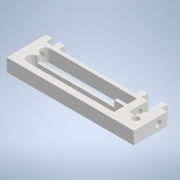
# Autodesk Inventor part: bottom slot
Saved by Autodesk Inventor 2020 (Build 240168000, 168)
## iProperties
Created: 2019-11-08
Part Number: bottom slot
Material: Generic
Document SubType Name: Modeling
Designer: Hymowitz
Density: 1 g/cm^3
Appearance: Default
Author: Hymowitz
## iProperties of the stored document _3DPrint.ipt
Created: 2019-11-25
Part Number: _3DPrint
Material: Generic
Document SubType Name: Modeling
Designer: Hymowitz
Density: 1 g/cm^3
Appearance: Default
Author: Hymowitz
Autodesk Inventor part; units mm, degrees
ref_plane "YZ Plane" through (0, 0, 0) normal (1, 0, 0) x (0, 1, 0)
ref_plane "XZ Plane" through (0, 0, 0) normal (0, 1, 0) x (-1, 0, 0)
ref_plane "XY Plane" through (0, 0, 0) normal (0, 0, 1) x (1, 0, 0)
sketch "Sketch1" plane through (0, 0, 0) normal (0, 1, 0) x (-1, 0, 0)
  line L0 (31.75, -3.048) -> (-31.75, -3.048)
  line L1 (-31.75, -3.048) -> (-31.75, 0)
  line L2 (-31.75, 0) -> (31.75, 0)
  line L3 (31.75, 0) -> (31.75, -3.048)
  line L4 (-31.75, 0) -> (31.75, 0)
  line L5 (31.75, 0) -> (31.75, 16.5722)
  line L6 (31.75, 16.5722) -> (-31.75, 16.5722)
  line L7 (-31.75, 16.5722) -> (-31.75, 0)
  line L8 (24.7167, 10.8097) -> (-19.6375, 10.8097) construction
  line L9 (24.7167, 13.3972) -> (-19.6375, 13.3972)
  line L10 (-19.6375, 8.2222) -> (24.7167, 8.2222)
  arc A0 (24.7167, 8.2222) -> (24.7167, 13.3972) centre (24.7167, 10.8097) ccw
  arc A1 (-19.6375, 13.3972) -> (-19.6375, 8.2222) centre (-19.6375, 10.8097) ccw
  line L11 (24.7167, 4.2534) -> (-24.7167, 4.2534) construction
  line L12 (24.7167, 6.6347) -> (-24.7167, 6.6347)
  line L13 (-24.7167, 1.8722) -> (24.7167, 1.8722)
  arc A2 (24.7167, 1.8722) -> (24.7167, 6.6347) centre (24.7167, 4.2534) ccw
  arc A3 (-24.7167, 6.6347) -> (-24.7167, 1.8722) centre (-24.7167, 4.2534) ccw
  line L14 (0, 0) -> (0, 22.7513) construction
  circle A4 centre (-26.9875, 10.8097) radius 1.5875
  point P0 (0, 4.2534)
  dimension "d5" = 49.4334
  dimension "d6" = 5.175
  dimension "d7" = 4.7625
  dimension "d8" = 4.2534
  dimension "d23" = 7.0333
  dimension "d24" = 3.175
  dimension "d25" = 3.175
  dimension "d26" = 3.175
  dimension "d27" = 1.5875
  dimension "d28" = 3.175
  constraints: 34 end point, 8 point on circle, 8 tangent, 5 centre point, 5 horizontal, 4 parallel, 3 vertical, 2 point on line, 1 collinear, 1 midpoint, 1 perpendicular, 4 other
  measures "d5" distance of L11.start L11.end
  measures "d6" distance between parallel lines of L9 L10
  measures "d7" distance between parallel lines of L13 L12
  measures "d8" distance between parallel lines of L2 L11
  measures "d23" distance from line of L5 L8.start
  measures "d24" diameter of A4
  measures "d25" distance edge to line of A4 L7
  measures "d27" distance between parallel lines of L12 L10
  measures "d28" distance between parallel lines of L6 L9
extrude "Extrusion1" add sketch "Sketch1" along normal mid plane 6.35 contours L2 L7 L6 L5
sketch "Sketch3" plane through (0, 3.175, 0) normal (0, 1, 0) x (1, 0, 0)
  arc A0 (24.7167, -6.6347) -> (24.7167, -1.8722) centre (24.7167, -4.2534) ccw projected
  line L0 (24.7167, -4.2534) -> (4.7773, -4.2534) construction
  line L1 (26.045, -9.5942) -> (22.235, -9.5942)
  line L2 (22.235, -9.5942) -> (22.235, 1.0874)
  line L3 (22.235, 1.0874) -> (26.045, 1.0874)
  line L4 (26.045, 1.0874) -> (26.045, -9.5942)
  line L5 (26.045, -9.5942) -> (22.235, 1.0874) construction
  line L6 (22.235, -9.5942) -> (26.045, 1.0874) construction
  point P0 (0, 0)
  point P1 (24.14, -4.2534)
  dimension "d14" = 10.6816
  dimension "d15" = 3.81
  constraints: 14 end point, 2 horizontal, 2 midpoint, 2 parallel, 1 perpendicular, 1 point on line
  measures "d14" distance of L3.end L1.start
  measures "d15" distance of L1.start L1.end
extrude "Extrusion3" cut sketch "Sketch3" against normal through all contours L4 L1 L2 L3
sketch "Sketch4" plane through (0, 3.175, 0) normal (0, 1, 0) x (1, 0, 0)
  line L0 (22.235, -6.6347) -> (-24.7167, -6.6347) projected
  line L1 (22.235, -1.8722) -> (-24.7167, -1.8722) projected
  line L2 (22.235, -6.6347) -> (18.6822, -6.6347)
  line L3 (18.6822, -6.6347) -> (18.6822, -1.8722)
  line L4 (18.6822, -1.8722) -> (22.235, -1.8722)
  line L5 (22.235, -1.8722) -> (22.235, -6.6347)
  point P0 (0, 0)
  point P1 (22.235, -1.8722)
  point P2 (18.6822, -6.6347)
  constraints: 8 end point, 2 parallel, 1 horizontal, 1 perpendicular, 1 point on line
extrude "Extrusion4" add sketch "Sketch4" against normal up to surface (6.35 mm away)
sketch "Sketch2" plane through (31.75, -3.175, 0) normal (1, 0, 0) x (0, 0, -1)
  line L0 (0, 3.175) -> (-16.5722, 3.175) construction
  line L1 (-16.5722, 6.35) -> (-16.5722, 0) construction
  line L2 (-6.6347, 0) -> (-6.6347, 6.35) construction
  line L3 (-1.8722, 6.35) -> (-1.8722, 0) construction
  circle A0 centre (-4.2534, 3.175) radius 1.5875
  line L4 (-6.6347, 0) -> (-6.6347, 6.35) construction
  line L5 (-6.6347, -1.3931) -> (-4.2534, -1.3931) construction
  line L6 (-1.8722, 0) -> (-1.8722, 6.35) construction
  line L7 (-1.8722, -1.3931) -> (-4.2534, -1.3931) construction
  line L8 (-4.2534, -1.3931) -> (-4.2534, 6.8506) construction
  line L9 (-6.6347, 6.35) -> (-6.6347, 0) projected
  line L10 (-1.8722, 0) -> (-1.8722, 6.35) projected
  point P0 (-7.4284, 6.35)
  point P1 (-7.4284, 0)
  dimension "d9" = 3.175
  constraints: 8 end point, 4 point on line, 1 centre point, 1 collinear, 1 horizontal, 1 midpoint, 1 perpendicular, 1 vertical, 2 other
  measures "d9" diameter of A0
extrude "Extrusion2" cut sketch "Sketch2" against normal through all
sketch "Sketch5" plane through (-24.7167, 3.175, 8.2222) normal (0, 0, 1) x (1, 0, 0)
  line L0 (24.7167, -3.175) -> (0, -3.175) construction
  line L1 (0, -6.35) -> (0, 0) construction
  line L2 (38.3736, -3.175) -> (0, -3.175)
  line L3 (0, -3.175) -> (0, 0)
  line L4 (0, 0) -> (38.3736, 0)
  line L5 (38.3736, 0) -> (38.3736, -3.175)
  line L6 (38.3736, -3.175) -> (0, 0) construction
  line L7 (0, -3.175) -> (38.3736, 0) construction
  line L8 (0, -6.35) -> (43.3989, -6.35) projected
  line L9 (43.3989, 0) -> (0, 0) projected
  point P0 (0, -3.175)
  dimension "d18" = 3.175
  dimension "d44" = 38.3736
  constraints: 14 end point, 3 point on line, 2 parallel, 1 collinear, 1 horizontal, 1 midpoint, 1 perpendicular
  measures "d18" distance between parallel lines of L4 L2
  measures "d44" distance of L3.end L4.end
extrude "Extrusion5" cut sketch "Sketch5" against normal up to next
sketch "Sketch6" plane through (31.75, -3.175, 0) normal (0, 0, -1) x (-1, 0, 0)
  line L0 (0, 7.366) -> (0, -4.826) projected
  line L1 (0, 6.35) -> (5.705, 6.35) projected
  line L2 (5.705, 0) -> (5.705, 6.35) projected
  line L3 (5.705, 0) -> (0, 0) projected
  line L4 (9.515, 6.35) -> (9.515, 0) projected
  line L5 (63.5, 0) -> (9.515, 0) projected
  line L6 (9.515, 0) -> (15.865, 0)
  line L7 (15.865, 0) -> (15.865, 6.35)
  line L8 (15.865, 6.35) -> (9.515, 6.35)
  line L9 (9.515, 6.35) -> (9.515, 0)
  line L10 (2.8525, 0) -> (2.8525, 6.35)
  line L11 (12.69, 0) -> (12.69, 6.35)
  line L12 (9.515, 6.35) -> (63.5, 6.35) projected
  line L13 (63.5, 0) -> (63.5, 6.35) projected
  line L14 (63.5, 0) -> (60.325, 0)
  line L15 (60.325, 0) -> (60.325, 6.35)
  line L16 (60.325, 6.35) -> (63.5, 6.35)
  line L17 (63.5, 6.35) -> (63.5, 0)
  line L18 (57.15, 0) -> (53.975, 0)
  line L19 (53.975, 0) -> (53.975, 6.35)
  line L20 (53.975, 6.35) -> (57.15, 6.35)
  line L21 (57.15, 6.35) -> (57.15, 0)
  point P0 (31.75, 3.175)
  point P1 (15.865, 0)
  point P2 (12.69, 0)
  dimension "d37" = 3.175
  dimension "d38" = 3.175
  dimension "d39" = 3.175
  dimension "d40" = 3.175
  dimension "d41" = 3.175
  constraints: 28 end point, 6 parallel, 5 perpendicular, 4 midpoint, 4 point on line, 3 horizontal, 1 collinear
  measures "d37" distance between parallel lines of L11 L7
  measures "d38" distance between parallel lines of L4 L11
  measures "d39" distance between parallel lines of L17 L15
  measures "d40" distance between parallel lines of L21 L15
  measures "d41" distance between parallel lines of L21 L19
extrude "Extrusion6" add sketch "Sketch6" along normal blind 3.175 contours L1 L2 L3 L10 | L8 L7 L5 L11 | L12 L21 L5 L19 | L12 L13 L5 L15
sketch "Sketch7" plane through (31.75, -3.175, 16.5722) normal (1, 0, 0) x (0, 0, -1)
  circle A0 centre (18.1597, 3.175) radius 0.75
  line L0 (16.5722, 3.175) -> (19.7472, 3.175)
  line L1 (16.5722, 0) -> (0, 0) projected
  line L2 (0, 6.35) -> (16.5722, 6.35) projected
  line L3 (19.7472, 6.35) -> (19.7472, 0) projected
  dimension "d32" = 1.5
  dimension "d33" = 1.5875
  constraints: 2 end point, 2 midpoint, 1 centre point, 1 horizontal
  measures "d32" diameter of A0
  measures "d33" distance of L0.end A0.centre
extrude "Extrusion7" cut sketch "Sketch7" against normal through all
sketch "Sketch8" plane through (0, -3.175, 0) normal (0, -1, 0) x (1, 0, 0)
  line L0 (22.235, 0) -> (22.235, 9.5942) projected
  line L1 (22.235, 9.5942) -> (25.9663, 9.5942) projected
  arc A0 (26.045, 9.5323) -> (25.9663, 9.5942) centre (26.9875, 10.8097) ccw projected
  line L2 (26.045, 9.5323) -> (26.045, 6.2298) projected
  arc A1 (26.045, 2.277) -> (26.045, 6.2298) centre (24.7167, 4.2534) ccw projected
  line L3 (26.045, 2.277) -> (26.045, -3.175) projected
  line L4 (28.8975, -3.175) -> (26.045, -3.175) projected
  line L5 (28.8975, 0) -> (28.8975, -3.175) projected
  line L6 (28.8975, 0) -> (31.75, 0) projected
  line L7 (31.75, 0) -> (31.75, 16.5722) projected
  line L8 (31.75, 16.5722) -> (-31.75, 16.5722) projected
  line L9 (-31.75, 16.5722) -> (-31.75, -3.175) projected
  line L10 (-28.575, -3.175) -> (-31.75, -3.175) projected
  line L11 (-28.575, 0) -> (-28.575, -3.175) projected
  line L12 (-28.575, 0) -> (-25.4, 0) projected
  line L13 (-25.4, 0) -> (-25.4, -3.175) projected
  line L14 (-22.225, -3.175) -> (-25.4, -3.175) projected
  line L15 (-22.225, 0) -> (-22.225, -3.175) projected
  line L16 (-22.225, 0) -> (15.885, 0) projected
  line L17 (15.885, 0) -> (15.885, -3.175) projected
  line L18 (19.06, -3.175) -> (15.885, -3.175) projected
  line L19 (19.06, 0) -> (19.06, -3.175) projected
  line L20 (19.06, 0) -> (22.235, 0) projected
  line L21 (-24.7167, 13.3972) -> (19.6375, 13.3972) projected
  arc A2 (19.6375, 8.2222) -> (19.6375, 13.3972) centre (19.6375, 10.8097) ccw projected
  line L22 (19.6375, 8.2222) -> (-24.7167, 8.2222) projected
  arc A3 (-24.7167, 13.3972) -> (-24.7167, 8.2222) centre (-24.7167, 10.8097) ccw projected
  line L23 (18.6822, 6.6347) -> (18.6822, 1.8722) projected
  line L24 (18.6822, 1.8722) -> (-24.7167, 1.8722) projected
  arc A4 (-24.7167, 6.6347) -> (-24.7167, 1.8722) centre (-24.7167, 4.2534) ccw projected
  line L25 (-24.7167, 6.6347) -> (18.6822, 6.6347) projected
  line L26 (19.6375, 8.2222) -> (-24.7167, 8.2222) projected
  line L27 (18.6822, 8.2222) -> (18.6822, 13.3972)
  point P0 (0, 0)
  constraints: 2 end point, 2 point on line, 1 collinear, 1 vertical
extrude "Extrusion8" add sketch "Sketch8" against normal blind 6.35 contours L21 A2 L22 L27
body "Solid1"
